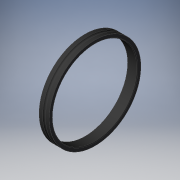
# Autodesk Inventor part: SKF_W 61710_ir
Saved by Autodesk Inventor 2019 (Build 230136000, 136)
## iProperties
Created: 2023-04-14
Part Number: SKF_W 61710_ir
Material: Generic
Catalog Web Link: www.cadenas.de
Description: BB1_001_101_ir-Deep groove ball bearings
Vendor: SKF
Document SubType Name: Modeling
Designer: psAdmin
Manufacturer: SKF
Mass: 2.04079 g
Surface Area: 26.4938 cm^2
Volume: 2.04079 cm^3
Density: 1 g/cm^3
Appearance: PSOLRGB-175-175-175
Category: PARTsolutions
Company: SKF
Title: SKF_W 61710_ir
Author: Cadenas PARTsolutions
Comments: Deep groove ball bearings
PSOL_IDENT_0: {$CADENAS_DATA/23d-libs/skf/bearings_units_and_housings/ball_bearings/deep_groove_ball_bearings/part
PSOL_IDENT_1: s/bb1_001_101_ir.prj},179 {VTYP=3D},{NB=SKF_W 61710_ir},{LINA=SKF_W 61710_ir},{NN=BB1_001_101_ir},{D
PSOL_IDENT_2: ATE=25.11.2022 05:56:16},{GEOMDATE=21.11.2022 10:23:00},{VERSION=},{LINEID=17550},{WBVAR=},{WBNUMERI
PSOL_IDENT_3: C=}  {NB=SKF_W 61710_ir},{LINA=SKF_W 61710_ir},{KT=DUMMY},{DESIGNATION=W 61710},{R12=0.30},{DD=50.00
PSOL_IDENT_4: 0},{D=62.000},{B=6.000},{C=},{CX=},{CXX=},{CA=0.000},{XXVARIANT=},{XXDESIGN=Single row stainless ste
PSOL_IDENT_5: el},{XXSEALING=No seals},{DESIGN=dgbbrs},{DESIGNIR=dgbbw},{VARIANT=},{DD1=54.30},{DD2=},{DD2X=},{DD2
PSOL_IDENT_6: A=0.00},{D1=57.80},{D1X=0.00},{D2=59.2},{D2A=59.20},{D3=},{D3X=},{D3A=0.000},{D4=},{HH=0.000},{BB=0.
PSOL_IDENT_7: 000},{BBX=},{BBA=0.000},{FF=},{R0MAX=0.000},{R0=0.000},{PITCH=56.00},{DW=2.381},{DDAMIN=52.000},{DDA
PSOL_IDENT_8: MAX=0.000},{DDBMIN=0.000},{DDBMAX=0.000},{DBMIN=0.000},{DAMAX=60.000},{BBAMIN=0.000},{CAMAX=0.000},{
PSOL_IDENT_9: RAMAX=0.300},{LOAD1=1.530},{LOAD2=1.530},{LOAD3=0.067},{SPEED1=22000},{SPEED2=13000},{KR=0.015},{F0=
PSOL_IDENT_10: 9.200},{Z=30},{II=1},{MASS=0.033},{BEARING=W 61710},{RING=},{HELP=2.100},{HELP2=1.400},{DD1ALG=27.15
PSOL_IDENT_11: 0},{YALG=27.150},{PITCH1=56.000},{DW1=2.381},{YALG1=28.900},{HALG1=2.100},{SH=27.150},{CU=0.724},{HA
PSOL_IDENT_12: LG=2.15},{B1=0},{SHIELDHELP=1},{D4A=0.000},{FFA=0.000},{RS1=},{HELP3=0},{SUPPRESS=0}
NB: SKF_W 61710_ir
NN: BB1_001_101_ir
NT: Deep groove ball bearings
NBSYN: SKF_$DESIGNATION._ir
LINA: SKF_W 61710_ir
CATALOG: SKF
DESIGNATION: W 61710
R12: 0.3
DD: 50
D: 62
B: 6
XXDESIGN: Single row stainless steel
XXSEALING: No seals
DD1: 54.3
D1: 57.8
D1X: 0
D2: 59.2
HH: 0
BB: 0
R0MAX: 0
R0: 0
PITCH: 56
DW: 2.381
DDAMIN: 52
DDAMAX: 0
DDBMIN: 0
DDBMAX: 0
DBMIN: 0
DAMAX: 60
BBAMIN: 0
CAMAX: 0
RAMAX: 0.3
LOAD1: 1.53
LOAD2: 1.53
LOAD3: 0.067
SPEED1: 22000
SPEED2: 13000
KR: 0.015
F0: 9.2
Z: 30
II: 1
MASS: 0.033
BEARING: W 61710
HELP3: 0
SUPPRESS: 0
SUPPLIER: SKF
ARTICLENO: SKF_W 61710_ir
BOMINFO: SKF_W 61710_ir
CREATOR: CADENAS GmbH
Autodesk Inventor part; units mm, degrees
sketch "Sketch_10" plane through (0, 0, 0) normal (0, 0, 1) x (1, 0, 0)
  line L0 (50, 0) -> (-50, 0)
  line L1 (0, 27.09) -> (0, 25.3)
  arc A0 (0, 25.3) -> (0.3, 25) centre (0.3, 25.3) ccw
  line L2 (0.3, 25) -> (5.7, 25)
  arc A1 (5.7, 25) -> (6, 25.3) centre (5.7, 25.3) ccw
  line L3 (6, 25.3) -> (6, 27.09)
  arc A2 (6, 27.09) -> (5.94, 27.15) centre (5.94, 27.09) ccw
  line L4 (5.94, 27.15) -> (3.8335, 27.15)
  arc A3 (2.1665, 27.15) -> (3.8335, 27.15) centre (3, 28) ccw
  line L5 (2.1665, 27.15) -> (0.06, 27.15)
  arc A4 (0.06, 27.15) -> (0, 27.09) centre (0.06, 27.09) ccw
  constraints: 12 end point, 10 point on circle, 5 centre point
revolve "Revolution1" add sketch "Sketch_10" angle 360 about axis through (50, 0, 0) along (1, 0, 0)
ref_plane "ir_XY" through (0, 0, 0) normal (0, 0, 1) x (1, 0, 0)
ref_plane "ir_YZ" through (0, 0, 0) normal (1, 0, 0) x (0, 1, 0)
ref_plane "ir_ZX" through (0, 0, 0) normal (0, 1, 0) x (0, 0, 1)
body "Solid1"
